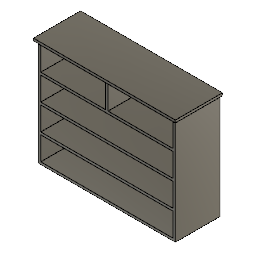
Dresser v4 (Autodesk Fusion 360 design; units mm, degrees)
Autodesk Fusion 360 part; units mm, degrees
sketch "Sketch1" plane through (0, 0, 0) normal (0, 0, 1) x (1, 0, 0)
  line L0 (550, 180) -> (-550, 180)
  line L1 (-550, 180) -> (-550, -180)
  line L2 (-550, -180) -> (550, -180)
  line L3 (550, -180) -> (550, 180)
  line L4 (550, 180) -> (-550, -180) construction
  line L5 (-550, 180) -> (550, -180) construction
  dimension "d1" = 1100
  dimension "d2" = 360
  constraint horizontal L0
  constraint perpendicular L0 L1
  constraint parallel L0 L2
  constraint parallel L1 L3
  constraint coincident L4 origin
  constraint coincident L5 origin
  measures "d1" distance of L1.end L2.end
  measures "d2" distance of L0.end L1.end
extrude "Extrude1" add sketch "Sketch1" along normal blind 850
sketch "Sketch2" plane through (0, 0, 850) normal (0, 0, 1) x (-1, 0, 0)
  line L0 (-550, -180) -> (550, -180)
  line L1 (550, -180) -> (570, -180)
  line L2 (-550, -180) -> (-570, -180)
  line L3 (-570, 180) -> (-570, 200)
  line L4 (-570, 200) -> (-550, 200)
  line L5 (570, -180) -> (-570, -180)
  line L6 (-570, -180) -> (-570, 200)
  line L7 (-570, 200) -> (570, 200)
  line L8 (570, 200) -> (570, -180)
  dimension "d5" = 20
  dimension "d7" = 20
  constraint coincident L0.end L1.start
  constraint coincident L0.start L2.start
  constraint vertical L3
  constraint horizontal L4
  constraint horizontal L5
  constraint vertical L6
  constraint horizontal L7
  constraint vertical L8
  measures "d5" distance of L0.end L1.end
  measures "d7" distance of L0.start L2.end
shell "Shell1" thickness 20 removed faces 1 at (-183.3333, -180, 283.3333)
extrude "Extrude2" add sketch "Sketch2" along normal blind 20
sketch "Sketch4" plane through (0, 160, 0) normal (0, -1, 0) x (1, 0, 0)
  line L0 (-530, 20) -> (530, 20)
  line L1 (530, 20) -> (530, 830)
  line L2 (530, 830) -> (-530, 830)
  line L3 (-530, 830) -> (-530, 20)
  line L4 (-530, 830) -> (-530, 642.5)
  line L5 (-530, 642.5) -> (530, 642.5)
  line L6 (530, 642.5) -> (530, 622.5)
  line L7 (530, 622.5) -> (-530, 622.5)
  line L8 (-530, 622.5) -> (-530, 642.5)
  line L9 (-530, 622.5) -> (-530, 435)
  line L10 (-530, 435) -> (530, 435)
  line L11 (530, 435) -> (530, 415)
  line L12 (530, 415) -> (-530, 415)
  line L13 (-530, 415) -> (-530, 435)
  line L14 (-530, 415) -> (-530, 227.5)
  line L15 (-530, 227.5) -> (530, 227.5)
  line L16 (530, 227.5) -> (530, 207.5)
  line L17 (530, 207.5) -> (-530, 207.5)
  line L18 (-530, 207.5) -> (-530, 227.5)
  dimension "d20" = 187.5
  dimension "d21" = 20
  dimension "d22" = 187.5
  dimension "d23" = 20
  dimension "d24" = 187.5
  dimension "d25" = 20
  constraint coincident L2.end L3.start
  constraint perpendicular L2 L4
  constraint horizontal L5
  constraint vertical L6
  constraint horizontal L7
  constraint vertical L8
  constraint perpendicular L7 L9
  constraint horizontal L10
  constraint vertical L11
  constraint horizontal L12
  constraint vertical L13
  constraint perpendicular L12 L14
  constraint horizontal L15
  constraint vertical L16
  constraint horizontal L17
  constraint vertical L18
  constraint coincident L1 L16.end
  measures "d20" distance of L2.end L4.end
  measures "d21" distance of L4.end L7.end
  measures "d22" distance of L7.end L9.end
  measures "d23" distance of L9.end L12.end
  measures "d24" distance of L12.end L14.end
  measures "d25" distance of L14.end L17.end
extrude "Extrude3" add sketch "Sketch4" along normal up to surface (340 mm away) contours L1 L3 L15 L16 L17 L18 | L1 L3 L10 L11 L12 L13 | L1 L3 L5 L6 L7 L8
sketch "Sketch5" plane through (0, 160, 0) normal (0, -1, 0) x (1, 0, 0)
  line L0 (-530, 642.5) -> (530, 642.5)
  line L1 (530, 642.5) -> (530, 830)
  line L2 (530, 830) -> (-530, 830)
  line L3 (-530, 830) -> (-530, 642.5)
  line L4 (0, 830) -> (-10, 830)
  line L5 (0, 642.5) -> (10, 642.5)
  line L6 (-10, 830) -> (10, 830)
  line L7 (10, 830) -> (10, 642.5)
  line L8 (10, 642.5) -> (-10, 642.5)
  line L9 (-10, 642.5) -> (-10, 830)
  dimension "d28" = 10
  dimension "d29" = 10
  constraint midpoint L2 L4.start
  constraint horizontal L4
  constraint midpoint L0 L5.start
  constraint horizontal L5
  constraint horizontal L6
  constraint vertical L7
  constraint horizontal L8
  constraint vertical L9
  measures "d28" distance of L4.start L4.end
  measures "d29" distance of L5.start L5.end
extrude "Extrude4" add sketch "Sketch5" along normal up to surface (340 mm away) contours L0 L2 L4 L5 L6 L7 L8 L9
